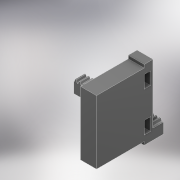
# Autodesk Inventor part: 6
Saved by Autodesk Inventor 2022 (Build 260153000, 153)
## iProperties
Company: HS Emden/Leer
Created: 2023-12-24
Part Number: 6
Material: PMMA-Kunststoff
Document SubType Name: Sheet Metal
Designer: Yaman Alsaady
Density: 1.188 g/cm^3
Appearance: Glatt - Schwarz
Sheet Metal Rule: Standard
Project: Delta-Robot
Author: Yaman Alsaady
Title: Rack
## iProperties of the stored document Rack_3D-Druck.ipt
Created: 2023-12-24
Part Number: Rack_3D-Druck
Material: Generisch
Document SubType Name: Modeling
Designer: alsaa
Density: 1 g/cm^3
Appearance: Vorgabe
Author: alsaa
Autodesk Inventor part; units mm, degrees
sketch "Skizze1" plane through (0, 0, 0) normal (0, 0, 1) x (1, 0, 0)
  line L0 (0, 0) -> (50.5, 0)
  line L1 (50.5, 0) -> (50.5, -6.5625)
  line L2 (50.5, -6.5625) -> (0, -6.5625)
  line L3 (0, -6.5625) -> (0, 0)
  line L4 (0.5, 0) -> (1.1142, 1.6875)
  line L5 (1.1142, 1.6875) -> (1.7463, 1.6875)
  line L6 (1.7463, 1.6875) -> (2.3605, 0)
  line L7 (1.4303, 1.6875) -> (1.4303, 0) construction
  line L8 (0.8412, 0.9375) -> (2.0193, 0.9375) construction
  dimension "d0" = 0.75
  dimension "d1" = 1.1781
  dimension "d2" = 20
  dimension "d3" = 1.6875
  dimension "d4" = 0.5
  dimension "d15" = 50
  dimension "d21" = 7.5
  constraints: 18 end point, 5 point on line, 3 perpendicular, 2 horizontal, 2 parallel, 1 coincident, 1 midpoint, 1 other
  measures "d0" distance between parallel lines of L5 L8
  measures "d1" distance of L8.start L8.end
  measures "d2" angle of L7 L4
  measures "d3" distance between parallel lines of L0 L5
  measures "d4" distance of L4.start L0.start
  measures "d15" distance of L0.end L4.start
  measures "d21" distance between parallel lines of L2 L8
extrude "Extrusion1" add sketch "Skizze1" along normal blind 6 contours L0 L1 L2 L3
extrude "Extrusion2" add sketch "Skizze1" along normal blind 6 contours L4 L5 L6 L0
fillet "Rundung1" radius 0.285 2 edges at (2.3605, 0, 3) (0.5, 0, 3)
pattern_linear "Rechteckige Anordnung1" count 21 spacing 2.3562 along (1, 0, 0) of "Rundung1", "Extrusion2"
sketch "Skizze2" plane through (0, -6.5625, 0) normal (-1, 0, 0) x (0, 0, 1)
  line L0 (0, 6.5625) -> (0, 0) projected
  line L1 (0, 0) -> (6, 0) projected
  line L2 (6, 6.5625) -> (6, 0) projected
  line L3 (0, 6.5625) -> (6, 6.5625) projected
extrude "Extrusion3" cut sketch "Skizze2" against normal up to surface (0.3004 mm away)
ref_plane "Arbeitsebene1" through (1.1142, 0.9375, 0) normal (0, 1, 0) x (1, 0, 0)
ref_plane "Arbeitsebene3" through (2.6084, 0, 6) normal (1, 0, 0) x (0, 1, 0)
ref_plane "Arbeitsebene2" through (1.4303, 1.6875, 6) normal (1, 0, 0) x (0, 1, 0)
sketch "Skizze4" plane through (0, 0, 6) normal (0, 0, 1) x (1, 0, 0)
  line L0 (0.3004, -6.5625) -> (50.5, -6.5625) projected
  line L1 (50.5, -6.5625) -> (40.5, -6.5625)
  line L2 (40.5, -6.5625) -> (40.5, 37.4375)
  line L3 (40.5, 37.4375) -> (50.5, 37.4375)
  line L4 (50.5, 37.4375) -> (50.5, -6.5625)
  point P0 (0, 0)
  dimension "d23" = 44
  dimension "d24" = 10
  constraints: 8 end point, 2 parallel, 1 horizontal, 1 perpendicular
  measures "d23" distance of L3.end L0.end
  measures "d24" distance between parallel lines of L4 L2
extrude "Extrusion5" add sketch "Skizze4" along normal blind 6
sketch "Skizze5" plane through (50.5, -6.5625, 0) normal (1, 0, 0) x (0, 0, -1)
  line L0 (-10, 27) -> (-6, 27)
  line L1 (-6, 27) -> (-6, 17)
  line L2 (-6, 17) -> (-10, 17)
  line L3 (-10, 17) -> (-10, 27)
  line L4 (-12, 44) -> (-12, 0) construction
  line L5 (-12, 22) -> (-6, 22) construction
  line L6 (-6, 6.5625) -> (-6, 44) construction
  point P0 (0, 6.5625)
  dimension "d27" = 4
  dimension "d28" = 10
  constraints: 10 end point, 2 horizontal, 2 midpoint, 2 parallel, 1 perpendicular, 1 point on line
  measures "d27" distance of L1.end L2.end
  measures "d28" distance of L2.end L0.start
extrude "Extrusion6" [suppressed]
ref_plane "Arbeitsebene4" through (16.7455, 0, 6) normal (1, 0, 0) x (0, 1, 0)
sketch "Skizze6" plane through (0, 0, 12) normal (0, 0, 1) x (1, 0, 0)
  line L0 (50.5, -4.5625) -> (40.5, -4.5625)
  line L1 (40.5, -4.5625) -> (40.5, 35.4375)
  line L2 (40.5, 35.4375) -> (50.5, 35.4375)
  line L3 (50.5, 35.4375) -> (50.5, -4.5625)
  line L4 (50.5, -6.5625) -> (50.5, 37.4375) projected
  line L5 (40.5, 37.4375) -> (40.5, -6.5625) projected
  point P0 (0, 0)
  point P1 (50.5, 15.4375)
  dimension "d31" = 40
  constraints: 8 end point, 2 midpoint, 2 parallel, 1 horizontal, 1 perpendicular, 1 point on line
  measures "d31" distance between parallel lines of L2 L0
extrude "Extrusion7" add sketch "Skizze6" along normal blind 30
sketch "Skizze7" plane through (0, 0, 6) normal (0, 0, -1) x (-1, 0, 0)
  line L0 (-40.5, 37.4375) -> (-40.5, 0.0392) projected
  line L1 (-50.5, 37.4375) -> (-40.5, 37.4375) projected
  line L2 (-50.5, 0) -> (-50.5, 37.4375) projected
  line L3 (-50.5, 0) -> (-50.5, 37.4375) projected
  line L4 (-50.5, 0) -> (-49.684, 0) projected
  line L5 (-47.4243, 0) -> (-47.3278, 0) projected
  line L6 (-45.0681, 0) -> (-44.9716, 0) projected
  line L7 (-42.7119, 0) -> (-42.6154, 0) projected
  line L8 (-40.5, 37.4375) -> (-40.5, 0.0392) projected
  arc A0 (-49.684, 0) -> (-49.4162, 0.1875) centre (-49.684, 0.285) ccw projected
  line L9 (-49.4162, 0.1875) -> (-48.8702, 1.6875) projected
  line L10 (-48.8702, 1.6875) -> (-48.2381, 1.6875) projected
  line L11 (-48.2381, 1.6875) -> (-47.6921, 0.1875) projected
  arc A1 (-47.6921, 0.1875) -> (-47.4243, 0) centre (-47.4243, 0.285) ccw projected
  arc A2 (-47.3278, 0) -> (-47.06, 0.1875) centre (-47.3278, 0.285) ccw projected
  line L12 (-47.06, 0.1875) -> (-46.514, 1.6875) projected
  line L13 (-46.514, 1.6875) -> (-45.8819, 1.6875) projected
  line L14 (-45.8819, 1.6875) -> (-45.3359, 0.1875) projected
  arc A3 (-45.3359, 0.1875) -> (-45.0681, 0) centre (-45.0681, 0.285) ccw projected
  arc A4 (-44.9716, 0) -> (-44.7038, 0.1875) centre (-44.9716, 0.285) ccw projected
  line L15 (-44.7038, 0.1875) -> (-44.1578, 1.6875) projected
  line L16 (-44.1578, 1.6875) -> (-43.5257, 1.6875) projected
  line L17 (-43.5257, 1.6875) -> (-42.9798, 0.1875) projected
  arc A5 (-42.9798, 0.1875) -> (-42.7119, 0) centre (-42.7119, 0.285) ccw projected
  arc A6 (-42.6154, 0) -> (-42.3476, 0.1875) centre (-42.6154, 0.285) ccw projected
  line L18 (-42.3476, 0.1875) -> (-41.8016, 1.6875) projected
  line L19 (-41.8016, 1.6875) -> (-41.1695, 1.6875) projected
  line L20 (-41.1695, 1.6875) -> (-40.6236, 0.1875) projected
  arc A7 (-40.6236, 0.1875) -> (-40.5, 0.0392) centre (-40.3557, 0.285) ccw projected
  line L21 (-50.5, 0) -> (-49.684, 0) projected
  arc A8 (-49.684, 0) -> (-49.4162, 0.1875) centre (-49.684, 0.285) ccw projected
  line L22 (-49.4162, 0.1875) -> (-48.8702, 1.6875) projected
  line L23 (-48.8702, 1.6875) -> (-48.2381, 1.6875) projected
  line L24 (-48.2381, 1.6875) -> (-47.6921, 0.1875) projected
  arc A9 (-47.6921, 0.1875) -> (-47.4243, 0) centre (-47.4243, 0.285) ccw projected
  line L25 (-47.4243, 0) -> (-47.3278, 0) projected
  arc A10 (-47.3278, 0) -> (-47.06, 0.1875) centre (-47.3278, 0.285) ccw projected
  line L26 (-47.06, 0.1875) -> (-46.514, 1.6875) projected
  line L27 (-46.514, 1.6875) -> (-45.8819, 1.6875) projected
  line L28 (-45.8819, 1.6875) -> (-45.3359, 0.1875) projected
  arc A11 (-45.3359, 0.1875) -> (-45.0681, 0) centre (-45.0681, 0.285) ccw projected
  line L29 (-45.0681, 0) -> (-44.9716, 0) projected
  arc A12 (-44.9716, 0) -> (-44.7038, 0.1875) centre (-44.9716, 0.285) ccw projected
  line L30 (-44.7038, 0.1875) -> (-44.1578, 1.6875) projected
  line L31 (-44.1578, 1.6875) -> (-43.5257, 1.6875) projected
  line L32 (-43.5257, 1.6875) -> (-42.9798, 0.1875) projected
  arc A13 (-42.9798, 0.1875) -> (-42.7119, 0) centre (-42.7119, 0.285) ccw projected
  line L33 (-42.7119, 0) -> (-42.6154, 0) projected
  arc A14 (-42.6154, 0) -> (-42.3476, 0.1875) centre (-42.6154, 0.285) ccw projected
  line L34 (-42.3476, 0.1875) -> (-41.8016, 1.6875) projected
  line L35 (-41.8016, 1.6875) -> (-41.1695, 1.6875) projected
  line L36 (-41.1695, 1.6875) -> (-40.6236, 0.1875) projected
  arc A15 (-40.6236, 0.1875) -> (-40.5, 0.0392) centre (-40.3557, 0.285) ccw projected
  line L37 (-50.5, 37.4375) -> (-40.5, 37.4375) projected
  point P0 (0, 0)
extrude "Extrusion8" [suppressed]
sketch "Skizze8" plane through (50.5, -6.5625, 0) normal (1, 0, 0) x (0, 0, -1)
  line L0 (-6, 44) -> (-12, 44) construction
  line L1 (-9, 44) -> (-9, 0) construction
  line L2 (0, 0) -> (-12, 0) construction
  line L3 (-9, 22) -> (-6, 22) construction
  line L4 (-6, 6.5625) -> (-6, 44) construction
  line L5 (-12, 30.5) -> (-8, 30.5)
  line L6 (-8, 30.5) -> (-8, 38.5)
  line L7 (-8, 38.5) -> (-12, 38.5)
  line L8 (-12, 38.5) -> (-12, 30.5)
  line L9 (-12, 42) -> (-42, 42) projected
  line L10 (-12, 13.5) -> (-8, 13.5)
  line L11 (-8, 13.5) -> (-8, 5.5)
  line L12 (-8, 5.5) -> (-12, 5.5)
  line L13 (-12, 5.5) -> (-12, 13.5)
  point P0 (0, 6.5625)
  point P1 (-8, 9.5)
  point P2 (-8, 34.5)
  dimension "d36" = 4
  dimension "d37" = 2
  dimension "d42" = 25
  dimension "d43" = 8
  constraints: 20 end point, 4 midpoint, 4 symmetric about line, 2 parallel, 2 perpendicular, 2 point on line, 1 horizontal, 1 vertical
  measures "d36" distance of L5.start L5.end
  measures "d37" distance between parallel lines of L4 L6
  measures "d42" distance of point (-8, 34.5) point (-8, 9.5)
  measures "d43" distance of L7.end L5.start
extrude "Extrusion9" cut sketch "Skizze8" against normal through all
sketch "Skizze9" plane through (0, 0, 6) normal (0, 0, -1) x (-1, 0, 0)
  line L0 (-50.5, 0) -> (-49.684, 0) projected
  arc A0 (-49.684, 0) -> (-49.4162, 0.1875) centre (-49.684, 0.285) ccw projected
  line L1 (-49.4162, 0.1875) -> (-48.8702, 1.6875) projected
  line L2 (-48.8702, 1.6875) -> (-48.2381, 1.6875) projected
  line L3 (-48.2381, 1.6875) -> (-47.6921, 0.1875) projected
  arc A1 (-47.6921, 0.1875) -> (-47.4243, 0) centre (-47.4243, 0.285) ccw projected
  line L4 (-47.4243, 0) -> (-47.3278, 0) projected
  arc A2 (-47.3278, 0) -> (-47.06, 0.1875) centre (-47.3278, 0.285) ccw projected
  line L5 (-47.06, 0.1875) -> (-46.514, 1.6875) projected
  line L6 (-46.514, 1.6875) -> (-45.8819, 1.6875) projected
  line L7 (-45.8819, 1.6875) -> (-45.3359, 0.1875) projected
  arc A3 (-45.3359, 0.1875) -> (-45.0681, 0) centre (-45.0681, 0.285) ccw projected
  line L8 (-45.0681, 0) -> (-44.9716, 0) projected
  arc A4 (-44.9716, 0) -> (-44.7038, 0.1875) centre (-44.9716, 0.285) ccw projected
  line L9 (-44.7038, 0.1875) -> (-44.1578, 1.6875) projected
  line L10 (-44.1578, 1.6875) -> (-43.5257, 1.6875) projected
  line L11 (-43.5257, 1.6875) -> (-42.9798, 0.1875) projected
  arc A5 (-42.9798, 0.1875) -> (-42.7119, 0) centre (-42.7119, 0.285) ccw projected
  line L12 (-42.7119, 0) -> (-42.6154, 0) projected
  arc A6 (-42.6154, 0) -> (-42.3476, 0.1875) centre (-42.6154, 0.285) ccw projected
  line L13 (-42.3476, 0.1875) -> (-41.8016, 1.6875) projected
  line L14 (-41.8016, 1.6875) -> (-41.1695, 1.6875) projected
  line L15 (-41.1695, 1.6875) -> (-40.6236, 0.1875) projected
  arc A7 (-40.6236, 0.1875) -> (-40.5, 0.0392) centre (-40.3557, 0.285) ccw projected
  line L16 (-40.5, 37.4375) -> (-40.5, 0.0392) projected
  line L17 (-50.5, 37.4375) -> (-40.5, 37.4375) projected
  line L18 (-50.5, 0) -> (-50.5, 37.4375) projected
  point P0 (0, 0)
extrude "Extrusion10" cut sketch "Skizze9" against normal blind 0.5
equation "\"d0\" = Module"
equation "\"d1\" = 1.5708 * Module"
equation "\"d2\" = Pressure_angle"
equation "\"d3\" = 2.25 * Module"
equation "\"d15\" = length"
equation "\"d11\" = 0.38 * Module"
equation "\"d14\" = 3.14159 * Module"
equation "\"Module\" = 0.75"
equation "\"Pressure_angle\" = 20deg"
equation "\"length\" = 50"
equation "\"d22\" = -Module"
equation "\"Biegeradius\" = Stärke"
equation "\"BreiteBiegungsfreistellung\" = Stärke"
equation "\"TiefeBiegungsfreistellung\" = 0.5 * Stärke"
equation "\"GrößeEckenfreistellung\" = 4 * Stärke"
equation "\"MinimalRest\" = 2 * Stärke"
equation "\"Übergangsradius\" = Biegeradius"
equation "\"JacobiRadiusGröße\" = Biegeradius"
equation "\"Abstandsgröße\" = Stärke"
equation "\"Stärke\" = 3.048"
